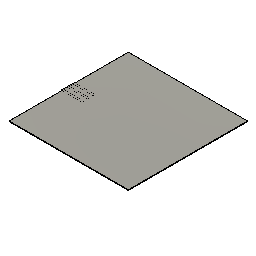
Platform (Autodesk Fusion 360 design; units mm, degrees)
Autodesk Fusion 360 part; units mm, degrees
sketch "Sketch1" plane through (0, 0, 0) normal (0, 1, 0) x (1, 0, 0)
  line L0 (0, 0) -> (1800, 0)
  line L1 (1800, 0) -> (1800, 1800)
  line L2 (1800, 1800) -> (0, 1800)
  line L3 (0, 1800) -> (0, 0)
  dimension "d1" = 1800
  dimension "d2" = 1800
  constraint horizontal L0
  constraint vertical L1
  constraint horizontal L2
  constraint vertical L3
  constraint coincident L0.start L3.end
  measures "d1" distance of L0.start L0.end
  measures "d2" distance of L0.start L2.end
extrude "Extrude1" add sketch "Sketch1" along normal blind 10 makes body 1
sketch "Sketch2" plane through (1800, 0, 0) normal (1, 0, 0) x (0, 0, -1)
  line L0 (0, 0) -> (1800, 0)
  line L1 (1800, 0) -> (1800, 10)
  line L2 (1800, 10) -> (0, 10)
  line L3 (0, 10) -> (0, 0)
  line L4 (800, 0) -> (1000, 0)
  line L5 (1000, 0) -> (1000, 190)
  line L6 (1000, 190) -> (800, 190)
  line L7 (800, 190) -> (800, 0)
  dimension "d5" = 200
  dimension "d6" = 190
  constraint horizontal L4
  constraint vertical L5
  constraint horizontal L6
  constraint vertical L7
  constraint coincident L0 L4.start
  constraint midpoint L0 L4
  measures "d5" distance of L4.start L4.end
  measures "d6" distance of L4.start L6.end
extrude "Extrude2" add sketch "Sketch2" along normal blind 10 contours L0 L2 L4 L5 L7 | L2 L5 L6 L7 bodies 1
sketch "Sketch3" plane through (0, 0, -800) normal (0, 0, 1) x (1, 0, 0)
  line L0 (1800, 190) -> (1800, 10)
  line L1 (1800, 10) -> (1800, 0)
  line L2 (1800, 0) -> (1810, 0)
  line L3 (1810, 0) -> (1810, 190)
  line L4 (1810, 190) -> (1800, 190)
  line L5 (1800, 190) -> (1785, 190)
  line L6 (1785, 190) -> (1785, 10)
  line L7 (1785, 10) -> (1800, 10)
  line L8 (1800, 10) -> (1800, 190)
  line L9 (1800, 10) -> (1500, 10)
  line L10 (1500, 10) -> (1500, 25)
  line L11 (1500, 25) -> (1800, 25)
  line L12 (1800, 25) -> (1800, 10)
  line L13 (1785, 145.8579) -> (1664.1421, 25)
  line L14 (1785, 160) -> (1650, 25)
  dimension "d9" = 15
  dimension "d10" = 15
  dimension "d11" = 180
  dimension "d12" = 300
  dimension "d13" = 45
  dimension "d14" = 10
  dimension "d15" = 30
  constraint horizontal L5
  constraint vertical L6
  constraint horizontal L7
  constraint vertical L8
  constraint coincident L0.start L4.end
  constraint horizontal L9
  constraint vertical L10
  constraint horizontal L11
  constraint vertical L12
  constraint coincident L0.end L1.start
  constraint coincident L6 L13.start
  constraint coincident L11 L13.end
  constraint coincident L6 L14.start
  constraint coincident L11 L14.end
  constraint parallel L13 L14
  measures "d9" distance of L9.end L10.end
  measures "d10" distance of L0.start L5.end
  measures "d11" distance of L5.end L6.end
  measures "d12" distance of L10.end L11.end
  measures "d13" angle of L11 L13
  measures "d14" distance of L13 L14
  measures "d15" distance of L5.end L14.start
extrude "Extrude3" add sketch "Sketch3" against normal blind 30 separate body contours L0 L5 L6 L8 L11 | L0 L6 L7 L8 L9 L11 L12 | L6 L9 L10 L11 | L6 L11 L13 L14 makes body 2
pattern_linear "R-Pattern1" count 3 spacing 85 along (0, 0, -1) of bodies 2 makes body 3 at (1645, 15, -885) makes body 4 at (1645, 15, -970)
combine "Combine1" operation add target body 1 tool bodies 2 3 4
move_body "Move1" bodies 1 to x (1, 0, 0) y (0, 1, 0) z (0, 0, 1) at (-905, 0, 900)
move_body "Move2" bodies 1 to x (-1, 0, 0) y (0, 0, -1) z (0, -1, 0) at (0, 0, 0)
scale "Scale1" [rolled back] scale factor 0.01
scale "Scale3" [rolled back] scale factor 0.1
